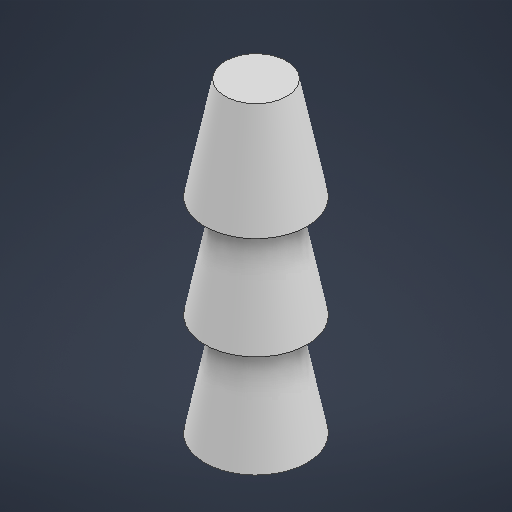
# Autodesk Inventor part: Valve_Plug_V2
Saved by Autodesk Inventor 2026.2 (Build 302298000, 298)
## iProperties
Created: 2026-01-25
Part Number: Valve_Plug_V2
Material: Generic
Document SubType Name: Modeling
Designer: vckot
Density: 1 g/cm^3
Appearance: Default
Author: vckot
Autodesk Inventor part; units mm, degrees
ref_plane "YZ Plane" through (0, 0, 0) normal (1, 0, 0) x (0, 1, 0)
ref_plane "XZ Plane" through (0, 0, 0) normal (0, 1, 0) x (-1, 0, 0)
ref_plane "XY Plane" through (0, 0, 0) normal (0, 0, 1) x (1, 0, 0)
sketch "Sketch1" plane through (0, 0, 0) normal (0, 0, 1) x (1, 0, 0)
  line L0 (-1.5, 0) -> (1.5, 0)
  line L1 (-2.5, -15) -> (2.5, -15)
  line L2 (-1.5, 0) -> (-2.5, -5)
  line L3 (1.5, 0) -> (2.5, -5)
  line L4 (1.5, -5) -> (1.5, -5)
  line L5 (-2.5, -10) -> (-1.5, -5)
  line L6 (1.5, -5) -> (2.5, -10)
  line L7 (-1.5, -10) -> (-1.5, -10)
  line L8 (1.5, -10) -> (2.5, -15)
  line L9 (-1.5, -10) -> (-2.5, -15)
  line L10 (1.5, -10) -> (2.5, -15)
  line L11 (0, 0) -> (0, -15)
  line L12 (-2.5, -10) -> (2.5, -10)
  line L13 (-2.5, -5) -> (2.5, -5)
  point P0 (0, -5)
  point P1 (0, -10)
  point P2 (0, -5)
  point P3 (0, -10)
  point P4 (1.9444, -10)
  dimension "d1" = 5
  dimension "d5" = 5
  dimension "d15" = 5
  dimension "d16" = 1.5
  dimension "d17" = 1.5
  dimension "d18" = 1.5
  dimension "d19" = 1.5
  dimension "d20" = 5
  dimension "d21" = 5
  dimension "d22" = 5
  constraints: 28 end point, 7 point on line, 4 midpoint, 3 horizontal, 3 vertical alignment, 2 parallel, 1 equal length, 1 vertical
  measures "d1" distance of L2.end L3.end
  measures "d5" distance of L1.start L1.end
  measures "d15" distance of L5.start L6.end
  measures "d16" distance from line of L11 L8.start
  measures "d17" distance from line of L11 L7.start
  measures "d18" distance from line of L11 L4.start
  measures "d19" distance from line of L11 L5.end
  measures "d20" distance between parallel lines of L0 L13
  measures "d21" distance between parallel lines of L13 L12
  measures "d22" distance between parallel lines of L12 L1
revolve "Revolution1" add sketch "Sketch1" angle 360 about axis through (0, 0, 0) along (0, -1, 0) contours L0 L3 L13 L11 | L13 L6 L12 L11 | L12 L8 L1 L11
body "Solid1"
